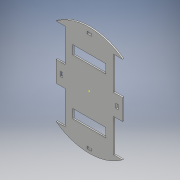
# Autodesk Inventor part: PakAnomRevisi
Saved by Autodesk Inventor 2017 (Build 210142000, 142)
## iProperties
Created: 2019-05-08
Part Number: PakAnomRevisi
Material: Generic
Document SubType Name: Modeling
Designer: Tio Refi
Density: 1 g/cm^3
Appearance: Default
Author: Tio Refi
Autodesk Inventor part; units mm, degrees
ref_plane "YZ Plane" through (0, 0, 0) normal (1, 0, 0) x (0, 1, 0)
ref_plane "XZ Plane" through (0, 0, 0) normal (0, 1, 0) x (-1, 0, 0)
ref_plane "XY Plane" through (0, 0, 0) normal (0, 0, 1) x (1, 0, 0)
sketch "Sketch1" plane through (0, 0, 0) normal (0, 1, 0) x (-1, 0, 0)
  line L0 (-75, 100) -> (-55, 100)
  line L1 (-55, 100) -> (-55, 25)
  line L2 (-55, 25) -> (-75, 25)
  line L3 (-75, 25) -> (-75, -22)
  line L4 (-75, -22) -> (-55, -22)
  line L5 (-55, -22) -> (-55, -97)
  line L6 (-55, -97) -> (-75, -97)
  line L7 (0, 0) -> (0, -13.688)
  line L8 (0, 0) -> (16.407, 0)
  line L9 (75, 100) -> (55, 100)
  line L10 (55, 100) -> (55, 25)
  line L11 (55, 25) -> (75, 25)
  line L12 (75, 25) -> (75, -22)
  line L13 (75, -22) -> (55, -22)
  line L14 (55, -22) -> (55, -97)
  line L15 (55, -97) -> (75, -97)
  arc A0 (75, 100) -> (-75, 100) centre (0, 0) ccw
  arc A1 (-75, -97) -> (75, -97) centre (0, 3) ccw
  line L16 (-60, -3.5) -> (-65, -3.5)
  line L17 (-65, -3.5) -> (-65, 6.5)
  line L18 (-65, 6.5) -> (-60, 6.5)
  line L19 (-60, 6.5) -> (-60, -3.5)
  line L20 (60, -3.5) -> (65, -3.5)
  line L21 (65, -3.5) -> (65, 6.5)
  line L22 (65, 6.5) -> (60, 6.5)
  line L23 (60, 6.5) -> (60, -3.5)
  constraints: 48 end point, 11 symmetric about line, 6 perpendicular, 6 point on line, 4 point on circle, 3 horizontal, 2 centre point, 2 parallel, 1 vertical
extrude "Extrusion1" add sketch "Sketch1" along normal mid plane 3 contours A0 L9 L10 L11 L12 L13 L14 L15 A1 L6 L5 L4 L3 L2 L1 L0 | L16 L17 L18 L19 | L23 L22 L21 L20
sketch "Sketch2" plane through (0, 1.5, 0) normal (0, 1, 0) x (1, 0, 0)
  point P0 (0, 0)
sketch "Sketch3" plane through (0, 1.5, 0) normal (0, 1, 0) x (1, 0, 0)
  line L0 (65, 3.5) -> (60, 3.5)
  line L1 (60, 3.5) -> (60, -6.5)
  line L2 (60, -6.5) -> (65, -6.5)
  line L3 (65, -6.5) -> (65, 3.5)
  line L4 (0, 0) -> (0, -6.5)
  line L5 (-65, 3.5) -> (-60, 3.5)
  line L6 (-60, 3.5) -> (-60, -6.5)
  line L7 (-60, -6.5) -> (-65, -6.5)
  line L8 (-65, -6.5) -> (-65, 3.5)
  constraints: 18 end point, 4 symmetric about line, 2 parallel, 1 horizontal, 1 perpendicular, 1 vertical
extrude "Extrusion2" cut sketch "Sketch3" against normal blind 3 contours L3 L2 L1 L0
sketch "Sketch4" plane through (0, -1.5, 0) normal (0, -1, 0) x (1, 0, 0)
  line L0 (-60, -3.5) -> (-65, -3.5)
  line L1 (-65, -3.5) -> (-65, 6.5)
  line L2 (-65, 6.5) -> (-60, 6.5)
  line L3 (-60, 6.5) -> (-60, -3.5)
  point P0 (0, 0)
  constraints: 8 end point, 2 parallel, 1 horizontal, 1 perpendicular
extrude "Extrusion3" cut sketch "Sketch4" against normal blind 3
sketch "Sketch5" plane through (0, -1.5, 0) normal (0, -1, 0) x (1, 0, 0)
  line L0 (-5, 110) -> (5, 110)
  line L1 (5, 110) -> (5, 115)
  line L2 (5, 115) -> (-5, 115)
  line L3 (-5, 115) -> (-5, 110)
  line L4 (0, 0) -> (8.5415, 0)
  line L5 (-5, -110) -> (5, -110)
  line L6 (5, -110) -> (5, -115)
  line L7 (5, -115) -> (-5, -115)
  line L8 (-5, -115) -> (-5, -110)
  constraints: 18 end point, 4 symmetric about line, 2 horizontal, 2 parallel, 1 perpendicular
extrude "Extrusion4" cut sketch "Sketch5" against normal blind 3
sketch "Sketch6" plane through (0, -1.5, 0) normal (0, -1, 0) x (1, 0, 0)
  line L0 (-37.5, 72.5) -> (37.5, 72.5)
  line L1 (37.5, 72.5) -> (37.5, 52.5)
  line L2 (37.5, 52.5) -> (-37.5, 52.5)
  line L3 (-37.5, 52.5) -> (-37.5, 72.5)
  line L4 (0, 0) -> (15.5313, 0)
  line L5 (-37.5, -72.5) -> (37.5, -72.5)
  line L6 (37.5, -72.5) -> (37.5, -52.5)
  line L7 (37.5, -52.5) -> (-37.5, -52.5)
  line L8 (-37.5, -52.5) -> (-37.5, -72.5)
  constraints: 18 end point, 4 symmetric about line, 2 horizontal, 2 parallel, 1 perpendicular
extrude "Extrusion5" cut sketch "Sketch6" against normal blind 3
sketch "Sketch7" plane through (0, -1.5, 0) normal (0, -1, 0) x (1, 0, 0)
  point P0 (0, 0)
sketch "Sketch8" plane through (0, -1.5, 0) normal (0, -1, 0) x (1, 0, 0)
  point P0 (0, 0)
body "Solid1"
